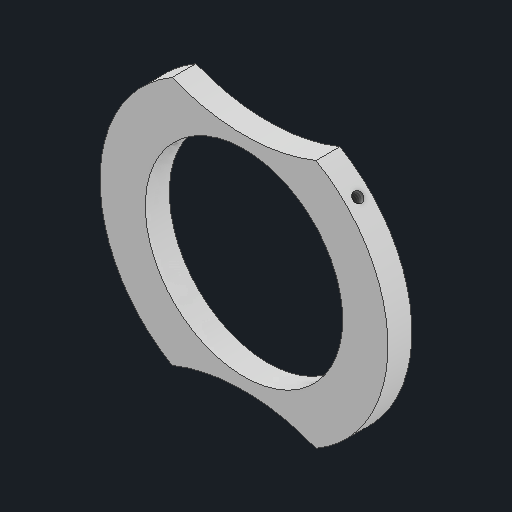
# Autodesk Inventor part: ShockCordSupportBulkhead
Saved by Autodesk Inventor 2026.2 (Build 302298010, 298A)
## iProperties
Created: 2026-03-08
Part Number: ShockCordSupportBulkhead
Material: Generic
Document SubType Name: Modeling
Designer: grhfa
Density: 1 g/cm^3
Appearance: Default
Author: grhfa
Autodesk Inventor part; units mm, degrees
ref_plane "XY Plane" through (0, 0, 0) normal (0, 0, 1) x (1, 0, 0)
sketch "Sketch1" plane through (0, 0, 0) normal (0, 0, 1) x (1, 0, 0)
  circle A0 centre (0, 0) radius 38.1
  arc A1 (-19.05, 32.9956) -> (19.05, 32.9956) centre (0, 80.0884) ccw
  line L0 (-38.1, 0) -> (38.1, 0) construction
  arc A2 (19.05, -32.9956) -> (-19.05, -32.9956) centre (0, -80.0884) ccw
  circle A3 centre (0, 0) radius 26.1134
  line L1 (0, 29.2884) -> (0, 26.1134) construction
  point P0 (-19.05, -32.9956)
  point P1 (19.05, -32.9956)
  dimension "d0" = 76.2
  dimension "d1" = 38.1
  dimension "d3" = 50.8
  dimension "d4" = 3.175
  constraints: 9 point on circle, 4 end point, 3 centre point, 3 symmetric about line, 2 coincident, 2 vertical alignment, 1 horizontal, 1 midpoint, 1 vertical, 3 other
  measures "d0" diameter of A0
  measures "d1" distance of A0.end A0.start
  measures "d3" radius of A1
  measures "d4" distance of L1.start L1.end
extrude "Extrusion1" add sketch "Sketch1" along normal mid plane 6.35 contours A0 A2 A1
ref_plane "Work Plane4" through (26.9408, -26.9408, 0) normal (-0.7071068, 0.7071068, 0) x (0, 0, 1)
ref_plane "Work Plane3" through (38.1, 38.1, 0) normal (-0.7071068, 0.7071068, 0) x (0, 0, 1)
sketch "Sketch2" plane through (26.9408, -26.9408, 0) normal (-0.7071068, 0.7071068, 0) x (0, 0, 1)
  point P0 (0, 0)
  point P1 (0, 0)
  constraints: 1 coincident
hole "Hole1" at (26.9408, -26.9408, 0) direction (-0.7071068, 0.7071068, 0) diameter 2.6416 depth 6.35 tip angle 118 thread size "6-32 UNC" class "2B" standard "ANSI Unified Screw Threads"
pattern_circular "Circular Pattern1" count 4 over 360 about axis through (0, 0, 0) along (0, 0, 1) of "Hole1"
ref_plane "Work Plane1" through (0, 38.1, 0) normal (0, 1, 0) x (-1, 0, 0)
ref_plane "Work Plane2" through (38.1, 0, 0) normal (1, 0, 0) x (0, 1, 0)
body "Solid1"
